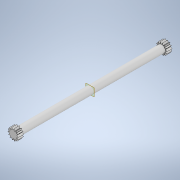
# Autodesk Inventor part: WelleRuder2
Saved by Autodesk Inventor 2021 (Build 250183000, 183)
## iProperties
Created: 2021-01-12
Part Number: WelleRuder2
Material: Generisch
Document SubType Name: Modeling
Designer: casa2
Density: 1 g/cm^3
Appearance: Vorgabe
Author: casa2
Autodesk Inventor part; units mm, degrees
ref_plane "YZ Plane" through (0, 0, 0) normal (1, 0, 0) x (0, 1, 0)
ref_plane "XZ Plane" through (0, 0, 0) normal (0, 1, 0) x (-1, 0, 0)
ref_plane "XY Plane" through (0, 0, 0) normal (0, 0, 1) x (1, 0, 0)
sketch "Skizze1" plane through (0, 0, 0) normal (0, 0, 1) x (1, 0, 0)
  circle A0 centre (0, 0) radius 5
  dimension "d0" = 10
  constraints: 1 centre point, 1 coincident
  measures "d0" diameter of A0
extrude "Extrusion1" add sketch "Skizze1" along normal blind 195
sketch "Skizze2" plane through (0, 0, 195) normal (0, 0, 1) x (1, 0, 0)
  circle A0 centre (0, 0) radius 5 projected
  circle A1 centre (0, 0) radius 7.5
  circle A2 centre (0, 0) radius 5 projected
  line L0 (0, -5) -> (-1.3746, -7.373)
  line L1 (-1.3746, -7.373) -> (-1.8625, -4.6402)
  arc A3 (-1.8625, -4.6402) -> (0, -5) centre (0, 0) ccw
  line L2 (2.1694, -4.5048) -> (1.9606, -7.2392)
  line L3 (1.9606, -7.2392) -> (0.3352, -4.9888)
  arc A4 (0.3352, -4.9888) -> (2.1694, -4.5048) centre (0, 0) ccw
  line L4 (3.9092, -3.1174) -> (4.9074, -5.6716)
  line L5 (4.9074, -5.6716) -> (2.4666, -4.3493)
  arc A5 (2.4666, -4.3493) -> (3.9092, -3.1174) centre (0, 0) ccw
  line L6 (4.8746, -1.1126) -> (6.8822, -2.9807)
  line L7 (6.8822, -2.9807) -> (4.1094, -2.8484)
  arc A6 (4.1094, -2.8484) -> (4.8746, -1.1126) centre (0, 0) ccw
  line L8 (4.8746, 1.1126) -> (7.494, 0.3005)
  line L9 (7.494, 0.3005) -> (4.9383, -0.7833)
  arc A7 (4.9383, -0.7833) -> (4.8746, 1.1126) centre (0, 0) ccw
  line L10 (3.9092, 3.1174) -> (6.6214, 3.5223)
  line L11 (6.6214, 3.5223) -> (4.7891, 1.4369)
  arc A8 (4.7891, 1.4369) -> (3.9092, 3.1174) centre (0, 0) ccw
  line L12 (2.1694, 4.5048) -> (4.4375, 6.0464)
  line L13 (4.4375, 6.0464) -> (3.6914, 3.3725)
  arc A9 (3.6914, 3.3725) -> (2.1694, 4.5048) centre (0, 0) ccw
  line L14 (0, 5) -> (1.3746, 7.373)
  line L15 (1.3746, 7.373) -> (1.8625, 4.6402)
  arc A10 (1.8625, 4.6402) -> (0, 5) centre (0, 0) ccw
  line L16 (-2.1694, 4.5048) -> (-1.9606, 7.2392)
  line L17 (-1.9606, 7.2392) -> (-0.3352, 4.9888)
  arc A11 (-0.3352, 4.9888) -> (-2.1694, 4.5048) centre (0, 0) ccw
  line L18 (-3.9092, 3.1174) -> (-4.9074, 5.6716)
  line L19 (-4.9074, 5.6716) -> (-2.4666, 4.3493)
  arc A12 (-2.4666, 4.3493) -> (-3.9092, 3.1174) centre (0, 0) ccw
  line L20 (-4.8746, 1.1126) -> (-6.8822, 2.9807)
  line L21 (-6.8822, 2.9807) -> (-4.1094, 2.8484)
  arc A13 (-4.1094, 2.8484) -> (-4.8746, 1.1126) centre (0, 0) ccw
  line L22 (-4.8746, -1.1126) -> (-7.494, -0.3005)
  line L23 (-7.494, -0.3005) -> (-4.9383, 0.7833)
  arc A14 (-4.9383, 0.7833) -> (-4.8746, -1.1126) centre (0, 0) ccw
  line L24 (-3.9092, -3.1174) -> (-6.6214, -3.5223)
  line L25 (-6.6214, -3.5223) -> (-4.7891, -1.4369)
  arc A15 (-4.7891, -1.4369) -> (-3.9092, -3.1174) centre (0, 0) ccw
  line L26 (-2.1694, -4.5048) -> (-4.4375, -6.0464)
  line L27 (-4.4375, -6.0464) -> (-3.6914, -3.3725)
  arc A16 (-3.6914, -3.3725) -> (-2.1694, -4.5048) centre (0, 0) ccw
  dimension "d3" = 15
  dimension "d6" = 360
  constraints: 56 end point, 30 point on circle, 14 centre point, 1 coincident, 1 concentric, 103 other
extrude "Extrusion2" add sketch "Skizze2" along normal blind 7 contours A0 | A0 L8 L9 | A0 L10 L11 | L6 L7 A0 | A0 L12 L13 | L4 L5 A0 | L15 A0 L14 | L3 A0 L2 | L17 A0 L16 | L1 A0 L0 | L19 A0 L18 | L27 A0 L26 | L21 A0 L20 | L25 A0 L24 | L23 A0 L22
ref_plane "Arbeitsebene1" through (0, 0, 97.5) normal (0, 0, -1) x (-1, 0, 0)
mirror "Spiegeln2" about plane through (0, 0, 97.5) normal (0, 0, -1) of "Extrusion2"
equation "\"d0\" = Durchmesser3"
equation "\"d3\" = Durchmesser1"
equation "\"Durchmesser1\" = 15"
equation "\"Größe1\" = 7"
equation "\"Durchmesser2\" = 3"
equation "\"Durchmesser3\" = 10"
equation "\"Größe3\" = 3"
equation "\"Größe4\" = 15"
